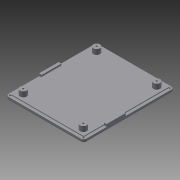
# Autodesk Inventor part: MotorDriverModel_lid
Saved by Autodesk Inventor 2015 (Build 190159000, 159)
## iProperties
Created: 2015-09-03
Part Number: MotorDriverModel_lid
Material: Generic
Document SubType Name: Modeling
Designer: Lauszus
Density: 1 g/cm^3
Appearance: Default
Author: Lauszus
Autodesk Inventor part; units mm, degrees
ref_plane "YZ Plane" through (0, 0, 0) normal (1, 0, 0) x (0, 1, 0)
ref_plane "XZ Plane" through (0, 0, 0) normal (0, 1, 0) x (-1, 0, 0)
ref_plane "XY Plane" through (0, 0, 0) normal (0, 0, 1) x (1, 0, 0)
sketch "Sketch1" plane through (0, 0, 0) normal (0, 1, 0) x (-1, 0, 0)
  line L0 (53.4667, 48.2438) -> (-53.5333, 48.2438)
  line L1 (-53.5333, 48.2438) -> (-53.5333, -43.7562)
  line L2 (-53.5333, -43.7562) -> (53.4667, -43.7562)
  line L3 (53.4667, -43.7562) -> (53.4667, 48.2438)
  point P0 (0, 0)
  dimension "d0" = 92
  dimension "d1" = 107
  constraints: 8 end point, 2 parallel, 1 horizontal, 1 perpendicular
  measures "d0" distance of L2.end L0.start
  measures "d1" distance of L1.end L2.end
extrude "Extrusion1" add sketch "Sketch1" along normal blind 3.5
sketch "Sketch3" plane through (0, 0, 0) normal (0, -1, 0) x (1, 0, 0)
  line L0 (50.3333, -40.5562) -> (-50.2667, -40.5562)
  line L1 (-50.2667, -40.5562) -> (-50.2667, 45.0438)
  line L2 (-50.2667, 45.0438) -> (50.3333, 45.0438)
  line L3 (50.3333, 45.0438) -> (50.3333, -40.5562)
  line L4 (53.5333, -43.7562) -> (-53.4667, -43.7562) projected
  line L5 (53.5333, 48.2438) -> (53.5333, -43.7562) projected
  line L6 (-53.4667, -43.7562) -> (-53.4667, 48.2438) projected
  line L7 (-53.4667, 48.2438) -> (53.5333, 48.2438) projected
  line L8 (-53.4667, 48.2438) -> (53.5333, 48.2438) projected
  line L9 (-12.9167, 45.0438) -> (10.4833, 45.0438)
  line L10 (10.4833, 48.2438) -> (-12.9167, 48.2438)
  point P0 (0, 0)
  dimension "d18" = 3.2
  dimension "d19" = 3.2
  dimension "d81" = 3.2
  dimension "d82" = 3.2
  constraints: 12 end point, 3 point on line, 2 collinear, 2 parallel, 1 horizontal, 1 perpendicular
  measures "d18" distance between parallel lines of L0 L4
  measures "d19" distance between parallel lines of L5 L3
  measures "d81" distance between parallel lines of L6 L1
  measures "d82" distance between parallel lines of L7 L2
extrude "Extrusion2" add sketch "Sketch3" along normal blind 1 contours L0 L1 L2 L3
sketch "Sketch4" plane through (0, -1, 0) normal (0, -1, 0) x (1, 0, 0)
  line L0 (50.3333, 45.0438) -> (-50.2667, 45.0438) projected
  line L1 (-43.4167, -33.3562) -> (43.4833, -33.3562)
  line L2 (43.4833, -33.3562) -> (43.4833, 37.8438)
  line L3 (43.4833, 37.8438) -> (-43.4167, 37.8438)
  line L4 (-43.4167, 37.8438) -> (-43.4167, -33.3562)
  line L5 (-50.2667, 45.0438) -> (-50.2667, -40.5562) projected
  line L6 (-50.2667, -40.5562) -> (50.3333, -40.5562) projected
  circle A0 centre (-43.4167, -33.3562) radius 4
  circle A1 centre (-43.4167, 37.8438) radius 4
  circle A2 centre (43.4833, 37.8438) radius 4
  circle A3 centre (43.4833, -33.3562) radius 4
  point P0 (0, 0)
  dimension "d24" = 71.2
  dimension "d25" = 86.9
  dimension "d26" = 6.85
  dimension "d27" = 7.2
  dimension "d28" = 8
  dimension "d29" = 8
  dimension "d30" = 8
  dimension "d31" = 8
  constraints: 8 end point, 4 centre point, 4 coincident, 2 parallel, 1 horizontal, 1 perpendicular
  measures "d24" distance of L1.end L2.end
  measures "d25" distance of L2.end L3.end
  measures "d26" distance between parallel lines of L4 L5
  measures "d27" distance between parallel lines of L6 L1
  measures "d28" diameter of A0
  measures "d29" diameter of A1
  measures "d30" diameter of A2
  measures "d31" diameter of A3
extrude "Extrusion3" add sketch "Sketch4" along normal blind 6 contours L4 A0 L1 | L1 A0 L4 | A3 L2 L1 | L1 L2 A3 | A1 L3 L4 | L4 L3 A1 | A2 L3 L2 | L2 L3 A2
sketch "Sketch2" plane through (0, 3.5, 0) normal (0, 1, 0) x (1, 0, 0)
  circle A0 centre (51.0333, -45.7438) radius 1
  line L0 (-53.4667, -48.2438) -> (53.5333, -48.2438) projected
  line L1 (53.5333, -48.2438) -> (53.5333, 43.7562) projected
  line L2 (0.0333, -35.8262) -> (0.0333, -54.6484)
  line L3 (-40.2723, -2.2438) -> (-66.6234, -2.2438)
  circle A1 centre (-50.9667, -45.7438) radius 1
  circle A2 centre (51.0333, 41.2562) radius 1
  circle A3 centre (-50.9667, 41.2562) radius 1
  point P0 (0, 0)
  dimension "d4" = 2
  dimension "d5" = 2.5
  dimension "d6" = 2.5
  dimension "d7" = 53.5
  dimension "d8" = 46
  constraints: 4 centre point, 4 end point, 3 symmetric about line, 1 horizontal, 1 vertical, 3 other
  measures "d4" diameter of A0
  measures "d5" distance from line of A0.centre L0
  measures "d6" distance from line of L1 A0.centre
  measures "d7" distance between parallel lines of L1 L2
  measures "d8" distance between parallel lines of L0 L3
hole "Hole1" at (51.0333, 3.5, 45.7438) at (-50.9667, 3.5, 45.7438) at (-50.9667, 3.5, -41.2562) at (51.0333, 3.5, -41.2562) direction (0, -1, 0) diameter 2 end through all countersink diameter 6 countersink angle 90
hole "Hole2" at (-43.4167, -7, 37.8438) direction (0, 1, 0) diameter 2 depth 9 tip angle 118
hole "Hole3" at (43.4833, -7, 37.8438) direction (0, 1, 0) diameter 2 depth 9 tip angle 118
hole "Hole4" at (43.4833, -7, -33.3562) direction (0, 1, 0) diameter 2 depth 9 tip angle 118
hole "Hole5" at (-43.4167, -7, -33.3562) direction (0, 1, 0) diameter 2 depth 9 tip angle 118
fillet "Fillet1" radius 3 4 edges at (-53.4667, 1.75, -43.7562) (53.5333, 1.75, -43.7562) (53.5333, 1.75, 48.2438) (-53.4667, 1.75, 48.2438)
fillet "Fillet2" radius 1 4 edges at (0.0333, 3.5, 48.2438) (53.5333, 3.5, 2.2438) (0.0333, 3.5, -43.7562) (-53.4667, 3.5, 2.2438)
sketch "Sketch7" plane through (0, 0, 0) normal (0, -1, 0) x (1, 0, 0)
  line L0 (-14.2167, 48.2438) -> (8.7833, 48.2438)
  line L1 (8.7833, 48.2438) -> (8.7833, 45.0438)
  line L2 (8.7833, 45.0438) -> (-14.2167, 45.0438)
  line L3 (-14.2167, 45.0438) -> (-14.2167, 48.2438)
  line L4 (-53.4667, -40.7562) -> (-53.4667, 45.2438) projected
  line L5 (50.3333, 45.0438) -> (-50.2667, 45.0438) projected
  point P0 (0, 0)
  dimension "d91" = 23
  dimension "d92" = 3.2
  dimension "d93" = 39.25
  dimension "d96" = 0
  constraints: 8 end point, 2 parallel, 1 horizontal, 1 perpendicular
  measures "d91" distance of L1.end L2.end
  measures "d92" distance of L2.end L0.start
  measures "d93" distance between parallel lines of L4 L3
  measures "d96" distance between parallel lines of L5 L2
extrude "Extrusion5" add sketch "Sketch7" along normal blind 3
sketch "Sketch8" plane through (0, 0, 0) normal (0, -1, 0) x (1, 0, 0)
  line L0 (-26.2167, -43.7562) -> (-3.7167, -43.7562)
  line L1 (-3.7167, -43.7562) -> (-3.7167, -40.5562)
  line L2 (-3.7167, -40.5562) -> (-26.2167, -40.5562)
  line L3 (-26.2167, -40.5562) -> (-26.2167, -43.7562)
  line L4 (-50.2667, -40.5562) -> (50.3333, -40.5562) projected
  line L5 (-53.4667, -40.7562) -> (-53.4667, 45.2438) projected
  point P0 (0, 0)
  dimension "d97" = 22.5
  dimension "d98" = 0
  dimension "d99" = 3.2
  dimension "d100" = 27.25
  constraints: 8 end point, 2 parallel, 1 horizontal, 1 perpendicular
  measures "d97" distance of L2.end L1.end
  measures "d98" distance between parallel lines of L2 L4
  measures "d99" distance of L0.end L1.end
  measures "d100" distance between parallel lines of L5 L3
extrude "Extrusion6" add sketch "Sketch8" along normal blind 3
body "Solid1"
